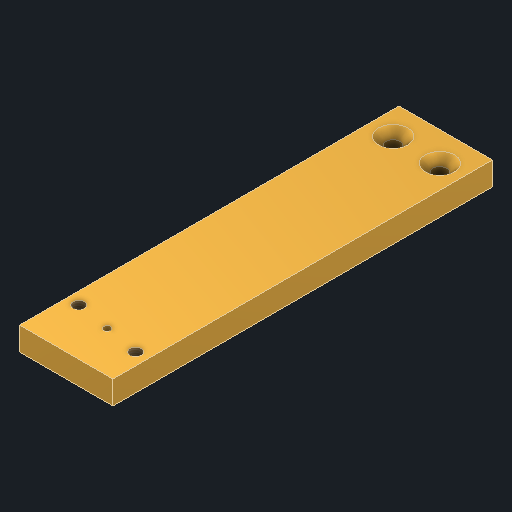
# Autodesk Inventor part: Support Beam
Saved by Autodesk Inventor 2027.1 (Build 311270010, 270A)
## iProperties
Created: 2025-09-16
Material: Brass, Soft Yellow
Document SubType Name: Modeling
Designer: SD
Density: 8.47 g/cm^3
Appearance: Brass - Satin
Mass: 460.823 g
Surface Area: 163.325 cm^2
Volume: 58.7035 cm^3
Project: Automatic Tea Steeping mechanism
Part Number: Support Beam
Length: 162.500 mm
Thickness: 10.000 mm
Width: 40.000 mm
BOM-Mass: 0.46082
BOM-Area: 0.016
Procurement: Fabricate - 1st round
Build Stage: 1
Preferred Material: C36000 Brass
Author: SD
Title: Support Beam
Autodesk Inventor part; units mm, degrees
ref_plane "YZ Plane" through (0, 0, 0) normal (1, 0, 0) x (0, 1, 0)
ref_plane "XZ Plane" through (0, 0, 0) normal (0, 1, 0) x (-1, 0, 0)
ref_plane "XY Plane" through (0, 0, 0) normal (0, 0, 1) x (1, 0, 0)
sketch "Sketch1" plane through (0, 0, 0) normal (0, 0, 1) x (1, 0, 0)
  line L0 (-20, 5) -> (20, 5)
  line L1 (20, 5) -> (20, -5)
  line L2 (20, -5) -> (-20, -5)
  line L3 (-20, -5) -> (-20, 5)
  line L4 (-20, 5) -> (20, -5) construction
  line L5 (20, 5) -> (-20, -5) construction
  point P0 (0, 0)
  constraints: 12 end point, 4 parallel, 2 midpoint, 1 horizontal, 1 perpendicular
extrude "Extrusion1" add sketch "Sketch1" along normal mid plane 162.5
sketch "Sketch4" plane through (-20, 5, 81.25) normal (0, 1, 0) x (1, 0, 0)
  line L0 (0, 162.5) -> (40, 162.5) projected
  point P0 (20, 81.25)
  point P1 (10, 150)
  point P2 (30, 150)
  dimension "d28" = 10
  dimension "d29" = 20
  dimension "d30" = 12.5
  constraints: 1 horizontal alignment
  measures "d28" horizontal distance of point (20, 81.25) point (10, 150)
  measures "d29" distance of point (30, 150) point (10, 150)
  measures "d30" distance from line of point (10, 150) L0
hole "Hole3" at (-10, 5, -68.75) at (10, 5, -68.75) direction (0, -1, 0) diameter 6 depth 10.4 countersink diameter 12.6 countersink angle 90
sketch "Sketch5" plane through (-20, 5, 81.25) normal (0, 1, 0) x (1, 0, 0)
  circle A0 centre (30, 150) radius 6.3 projected
  point P0 (20, 81.25)
  point P1 (20, 17.5)
  dimension "d38" = 132.5
  constraints: 1 vertical alignment
  measures "d38" vertical distance of point (20, 17.5) A0.centre
hole "Hole4" at (0, 5, 63.75) direction (0, -1, 0) diameter 3 depth 10.4
sketch "Sketch6" plane through (-20, 5, 81.25) normal (0, 1, 0) x (1, 0, 0)
  circle A0 centre (20, 17.5) radius 1.5 projected
  line L0 (20, 17.5) -> (3, 17.5) construction
  line L1 (5.23, 20.1043) -> (20, 17.5) construction
  line L2 (20, 17.5) -> (34.77, 14.8957) construction
  point P0 (20, 81.25)
  dimension "d46" = 10
  dimension "d47" = 10
  dimension "d48" = 14.77
  dimension "d49" = 14.77
  constraints: 6 end point, 1 coincident, 1 horizontal
  measures "d46" angle of L0 L1
  measures "d47" angle of L2 L0
  measures "d48" horizontal distance of L0.start L1.start
  measures "d49" horizontal distance of L2.end L0.start
hole "Hole5" at (-14.77, 5, 61.1457) at (14.77, 5, 66.3543) direction (0, -1, 0) diameter 4.917 depth 17.1 thread size "M6x1" class "6H" standard "ISO Metric profile"
equation "\"d49\" = d48"
body "Solid1"
